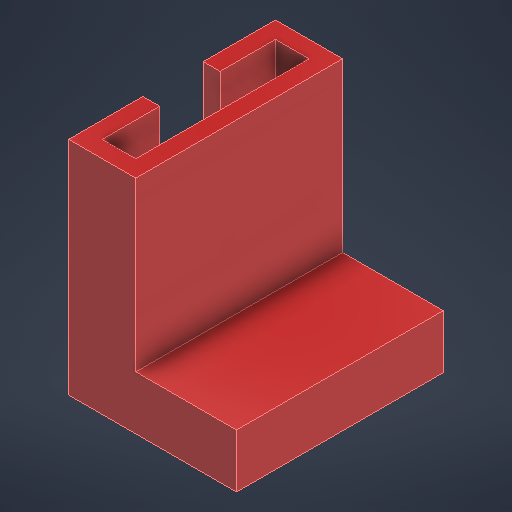
# Autodesk Inventor part: base camera
Saved by Autodesk Inventor 2026 (Build 300175000, 175)
## iProperties
Created: 2025-04-15
Part Number: base camera
Material: Generic
Document SubType Name: Modeling
Designer: ADM
Density: 1 g/cm^3
Appearance: Red
Author: ADM
Autodesk Inventor part; units mm, degrees
ref_plane "YZ Plane" through (0, 0, 0) normal (1, 0, 0) x (0, 1, 0)
ref_plane "XZ Plane" through (0, 0, 0) normal (0, 1, 0) x (-1, 0, 0)
ref_plane "XY Plane" through (0, 0, 0) normal (0, 0, 1) x (1, 0, 0)
sketch "Sketch1" plane through (0, 0, 0) normal (0, 1, 0) x (-1, 0, 0)
  line L0 (0, 0) -> (5, 0)
  line L1 (5, 0) -> (5, -25.8)
  line L2 (5, -25.8) -> (0, -25.8)
  line L3 (0, -25.8) -> (0, 0)
  line L4 (7.5, -28.3) -> (7.5, 2.5)
  line L5 (7.5, 2.5) -> (-2.5, 2.5)
  line L6 (-2.5, 2.5) -> (-2.5, -28.3)
  line L7 (-2.5, -28.3) -> (7.5, -28.3)
  dimension "d0" = 5
  dimension "d1" = 25.8
  dimension "d2" = 2.5
  constraints: 16 end point, 4 parallel, 2 perpendicular, 1 horizontal, 3 other
  measures "d0" distance of L1.end L2.end
  measures "d1" distance of L0.end L1.end
  measures "d2" distance between parallel lines of L1 L4
extrude "Extrusion1" add sketch "Sketch1" along normal blind 25
sketch "Sketch2" plane through (0, 0, 0) normal (0, -1, 0) x (1, 0, 0)
  line L0 (2.5, -28.3) -> (-7.5, -28.3) projected
  line L1 (-7.5, 2.5) -> (2.5, 2.5) projected
  line L2 (2.5, -28.3) -> (-7.5, -28.3)
  line L3 (-7.5, -28.3) -> (-7.5, 2.5)
  line L4 (-7.5, 2.5) -> (2.5, 2.5)
  line L5 (2.5, 2.5) -> (2.5, -28.3)
  point P0 (0, 0)
  point P1 (2.5, 2.5)
  constraints: 8 end point, 2 parallel, 1 horizontal, 1 perpendicular
extrude "Extrusion2" add sketch "Sketch2" along normal blind 8
sketch "Sketch3" plane through (2.5, 25, 2.5) normal (1, 0, 0) x (0, 0, -1)
  line L0 (30.8, -33) -> (0, -33) projected
  line L1 (0, -33) -> (0, 0) projected
  line L2 (30.8, -33) -> (0, -33)
  line L3 (0, -33) -> (0, -25)
  line L4 (0, -25) -> (30.8, -25)
  line L5 (30.8, -25) -> (30.8, -33)
  point P0 (2.5, -25)
  dimension "d7" = 8
  constraints: 8 end point, 2 parallel, 1 horizontal, 1 perpendicular, 1 point on line
  measures "d7" distance of L2.end L3.end
extrude "Extrusion3" add sketch "Sketch3" along normal blind 15
sketch "Sketch4" plane through (0, 25, 0) normal (0, 1, 0) x (1, 0, 0)
  line L0 (-5, 0) -> (-5, 25.8) projected
  line L1 (-7.5, -2.5) -> (-7.5, 28.3) projected
  line L2 (-5, 17.55) -> (-7.5, 17.55)
  line L3 (-7.5, 17.55) -> (-7.5, 8.55)
  line L4 (-7.5, 8.55) -> (-5, 8.55)
  line L5 (-5, 8.55) -> (-5, 17.55)
  line L6 (2.5, 28.3) -> (-7.5, 28.3) projected
  point P0 (0, 0)
  point P1 (-5, 8.55)
  point P2 (-7.5, 17.55)
  dimension "d10" = 9
  dimension "d11" = 10.75
  constraints: 8 end point, 2 parallel, 2 point on line, 1 horizontal, 1 perpendicular
  measures "d10" distance of L3.end L2.end
  measures "d11" distance between parallel lines of L6 L2
extrude "Extrusion4" cut sketch "Sketch4" against normal blind 15
body "Solid1"
